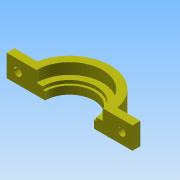
# Autodesk Inventor part: 电机座上轴盖
Saved by Autodesk Inventor 2015 (Build 190159000, 159)
## iProperties
Created: 2017-05-27
Part Number: 电机座上轴盖
Material: 常规
Document SubType Name: Modeling
Designer: Administrator
Density: 1 g/cm^3
Appearance: 黄色
Author: Administrator
Autodesk Inventor part; units mm, degrees
ref_plane "YZ Plane" through (0, 0, 0) normal (1, 0, 0) x (0, 1, 0)
ref_plane "XZ Plane" through (0, 0, 0) normal (0, 1, 0) x (-1, 0, 0)
ref_plane "XY Plane" through (0, 0, 0) normal (0, 0, 1) x (1, 0, 0)
sketch "草图1" plane through (0, 0, 0) normal (0, 0, 1) x (1, 0, 0)
  line L0 (-40, 0) -> (40, 0)
  line L1 (40, 0) -> (40, 5)
  line L2 (40, 5) -> (-40, 5)
  line L3 (-40, 5) -> (-40, 0)
  arc A0 (26, 0) -> (-26, 0) centre (0, 0) ccw
  dimension "d0" = 80
  dimension "d1" = 5
  dimension "d2" = 26
  constraints: 8 end point, 2 coincident, 2 parallel, 2 point on circle, 2 point on line, 1 centre point, 1 horizontal, 1 midpoint, 1 perpendicular
  measures "d0" distance of L2.end L1.end
  measures "d1" distance of L0.end L1.end
  measures "d2" radius of A0
extrude "拉伸1" add sketch "草图1" along normal blind 14
sketch "草图2" plane through (0, 0, 14) normal (0, 0, 1) x (1, 0, 0)
  circle A0 centre (0, 0) radius 21
  dimension "d5" = 42
  constraints: 1 centre point, 1 coincident
  measures "d5" diameter of A0
extrude "拉伸2" cut sketch "草图2" against normal blind 7
sketch "草图3" plane through (0, 0, 7) normal (0, 0, 1) x (1, 0, 0)
  circle A0 centre (0, 0) radius 17
  dimension "d8" = 34
  constraints: 1 centre point, 1 coincident
  measures "d8" diameter of A0
extrude "拉伸3" cut sketch "草图3" against normal blind 2
sketch "草图4" plane through (0, 0, 5) normal (0, 0, 1) x (1, 0, 0)
  circle A0 centre (0, 0) radius 15.5
  dimension "d11" = 31
  constraints: 1 centre point, 1 coincident
  measures "d11" diameter of A0
extrude "拉伸4" cut sketch "草图4" against normal blind 5
sketch "草图5" plane through (-40, 5, 0) normal (0, 1, 0) x (1, 0, 0)
  circle A0 centre (7, -7) radius 2.5
  circle A1 centre (73, -7) radius 2.5
  line L0 (80, 0) -> (80, -14) projected
  line L1 (80, -14) -> (65.5147, -14) projected
  line L2 (0, 0) -> (0, -14) projected
  line L3 (14.4853, -14) -> (0, -14) projected
  point P0 (40, 0)
  dimension "d14" = 5
  dimension "d15" = 5
  dimension "d16" = 7
  dimension "d17" = 7
  dimension "d18" = 7
  dimension "d19" = 7
  constraints: 2 centre point
  measures "d14" diameter of A0
  measures "d15" diameter of A1
  measures "d16" distance from line of A1.centre L0
  measures "d17" distance from line of A1.centre L1
  measures "d18" distance from line of L2 A0.centre
  measures "d19" distance from line of L3 A0.centre
extrude "拉伸5" cut sketch "草图5" against normal through all
